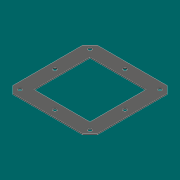
# Autodesk Inventor part: backplaneGasket
Saved by Autodesk Inventor 2016 SP1 (Build 200210100, 210)
## iProperties
Created: 2015-12-22
Part Number: backplaneGasket
Material: Rubber
Document SubType Name: Modeling
Designer: sawai
Density: 0.93 g/cm^3
Appearance: Rubber - Black
Author: sawai
Autodesk Inventor part; units mm, degrees
ref_plane "YZ Plane" through (0, 0, 0) normal (1, 0, 0) x (0, 1, 0)
ref_plane "XZ Plane" through (0, 0, 0) normal (0, 1, 0) x (-1, 0, 0)
ref_plane "XY Plane" through (0, 0, 0) normal (0, 0, 1) x (1, 0, 0)
sketch "Sketch1" plane through (0, 0, 0) normal (0, 0, 1) x (1, 0, 0)
  line L0 (-38.1, 38.1) -> (38.1, 38.1)
  line L1 (38.1, 38.1) -> (38.1, -38.1)
  line L2 (38.1, -38.1) -> (-38.1, -38.1)
  line L3 (-38.1, -38.1) -> (-38.1, 38.1)
  line L4 (-38.1, 38.1) -> (38.1, -38.1) construction
  line L5 (38.1, 38.1) -> (-38.1, -38.1) construction
  point P0 (0, 0)
  dimension "d0" = 76.2
  dimension "d1" = 76.2
  constraints: 12 end point, 2 midpoint, 2 parallel, 1 horizontal, 1 perpendicular
  measures "d0" distance of L1.end L2.end
  measures "d1" distance of L0.end L1.end
extrude "Extrusion1" add sketch "Sketch1" along normal blind 0.7937
sketch "Sketch2" plane through (0, 0, 0.7937) normal (0, 0, 1) x (1, 0, 0)
  line L0 (38.1, 38.1) -> (-38.1, 38.1) projected
  line L1 (-38.1, 38.1) -> (-38.1, -38.1) projected
  line L2 (-38.1, -38.1) -> (38.1, -38.1) projected
  line L3 (38.1, -38.1) -> (38.1, 38.1) projected
  line L4 (-31.75, 31.75) -> (31.75, 31.75)
  line L5 (31.75, 31.75) -> (31.75, -31.75)
  line L6 (31.75, -31.75) -> (-31.75, -31.75)
  line L7 (-31.75, -31.75) -> (-31.75, 31.75)
  point P0 (0, 0)
  point P1 (0, 31.75)
  point P2 (31.75, 0)
  point P3 (0, -31.75)
  point P4 (-31.75, 0)
  dimension "d7" = 6.35
  constraints: 8 end point, 4 coincident, 4 midpoint, 3 other
  measures "d7" distance between parallel lines of L0 L4
chamfer "Chamfer1" distance 6.35 angle 45 4 edges at (38.1, 38.1, 0.3969) (-38.1, 38.1, 0.3969) (38.1, -38.1, 0.3969) (-38.1, -38.1, 0.3969)
hole "Hole1" at (-31.75, 31.75, 0.7937) at (0, 31.75, 0.7937) at (31.75, 31.75, 0.7937) at (31.75, 0, 0.7937) at (31.75, -31.75, 0.7937) at (0, -31.75, 0.7937) at (-31.75, -31.75, 0.7937) at (-31.75, 0, 0.7937) direction (0, 0, -1) diameter 3.264 end through all clearance for "Hex Machine Screw" size "#4" standard "Ansi Unified Screw Threads"
sketch "Sketch3" plane through (0, 0, 0.7937) normal (0, 0, 1) x (1, 0, 0)
  line L0 (-25.4, -25.4) -> (25.4, -25.4)
  line L1 (25.4, -25.4) -> (25.4, 25.4)
  line L2 (25.4, 25.4) -> (-25.4, 25.4)
  line L3 (-25.4, 25.4) -> (-25.4, -25.4)
  line L4 (-25.4, -25.4) -> (25.4, 25.4) construction
  line L5 (25.4, -25.4) -> (-25.4, 25.4) construction
  point P0 (0, 0)
  dimension "d15" = 50.8
  dimension "d16" = 50.8
  constraints: 12 end point, 2 midpoint, 2 parallel, 1 horizontal, 1 perpendicular
  measures "d15" distance of L0.start L0.end
  measures "d16" distance of L0.end L1.end
extrude "Extrusion2" cut sketch "Sketch3" against normal through all
equation "\"d7\" = backplaneHoleOffsett"
equation "\"frameAcrylicThickness\" = 9.525"
equation "\"internalAcrylicThickness\" = 6.35"
equation "\"height\" = 127"
equation "\"width\" = 127"
equation "\"depth\" = 273.05"
equation "\"mirrorAngle\" = 5deg"
equation "\"detectorWidth\" = 52"
equation "\"detectorHeight\" = 52"
equation "\"mirrorThickness\" = 3.175"
equation "\"fresnelThickness\" = 0.1"
equation "\"focalLength\" = 76.2"
equation "\"ior\" = 1.49"
equation "\"centerThickness\" = 1.524"
equation "\"fresnelAngle\" = 90deg"
equation "\"fresnelEffectiveDiameter\" = 152.4"
equation "\"oRingWidth\" = 1.5875"
equation "\"sensorHolderDepth\" = 19.05"
equation "\"aerogelClearence\" = 3.175"
equation "\"backplanePCBWidth\" = 76.2"
equation "\"backplanePCBHeight\" = 76.2"
equation "\"backplaneHoleOffsett\" = 6.35"
equation "\"backplanePostionOffsett\" = 12.7"
equation "\"moduleSlotClearence\" = 0.79375"
body "Solid1"
